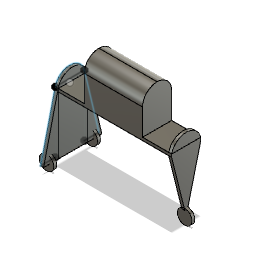
test_3 v2 (Autodesk Fusion 360 design; units mm, degrees)
part number: Configuration 1
Autodesk Fusion 360 part; units mm, degrees
sketch "Sketch1" plane through (0, 0, 0) normal (0, 0, 1) x (1, 0, 0)
  line L0 (0, 0) -> (200, 0)
  line L1 (200, 0) -> (200, 100)
  line L2 (200, 100) -> (0, 100)
  line L3 (0, 100) -> (0, 0)
  dimension "d1" = 200
  dimension "d2" = 100
  constraint horizontal L0
  constraint vertical L1
  constraint horizontal L2
  constraint vertical L3
  constraint coincident L0.start L3.end
  measures "d1" distance of L0.start L0.end
  measures "d2" distance of L0.start L2.end
extrude "Extrude1" add sketch "Sketch1" along normal blind 100 makes body 1
move_body "Move1" bodies 1 to x (1, 0, 0) y (0, 1, 0) z (0, 0, 1) at (0, 200, 0)
sketch "Sketch2" plane through (200, 0, 0) normal (1, 0, 0) x (0, 0, -1)
  line L0 (0, 200) -> (0, 300)
  line L1 (0, 300) -> (-100, 300)
  line L2 (-100, 300) -> (-100, 200)
  line L3 (-100, 200) -> (0, 200)
  line L4 (-100, 300) -> (-120, 300)
  line L5 (-120, 300) -> (-120, 280)
  line L6 (-120, 280) -> (-100, 280)
  line L7 (-100, 280) -> (-100, 300)
  line L8 (0, 300) -> (20, 300)
  line L9 (20, 300) -> (20, 280)
  line L10 (20, 280) -> (0, 280)
  line L11 (0, 280) -> (0, 300)
  dimension "d5" = 20
  dimension "d6" = 20
  dimension "d7" = 20
  dimension "d8" = 20
  constraint horizontal L4
  constraint vertical L5
  constraint horizontal L6
  constraint vertical L7
  constraint coincident L1.end L2.start
  constraint horizontal L8
  constraint vertical L9
  constraint horizontal L10
  constraint vertical L11
  constraint coincident L0.end L1.start
  measures "d5" distance of L1.end L4.end
  measures "d6" distance of L1.end L6.end
  measures "d7" distance of L0.end L8.end
  measures "d8" distance of L0.end L10.end
sketch "Sketch3" plane through (200, 0, 0) normal (1, 0, 0) x (0, 0, -1)
  line L0 (0, 200) -> (0, 300)
  line L1 (0, 300) -> (-100, 300)
  line L2 (-100, 300) -> (-100, 200)
  line L3 (-100, 200) -> (0, 200)
  line L4 (-100, 200) -> (0, 200)
  line L5 (0, 200) -> (0, 210)
  line L6 (0, 210) -> (-100, 210)
  line L7 (-100, 210) -> (-100, 200)
  dimension "d11" = 100
  dimension "d12" = 10
  constraint horizontal L4
  constraint vertical L5
  constraint horizontal L6
  constraint vertical L7
  constraint coincident L2.end L3.start
  measures "d11" distance of L2.end L0.start
  measures "d12" distance of L2.end L6.end
extrude "Extrude3" add sketch "Sketch3" along normal blind 100 separate body contours L0 L2 L3 L4 L5 L6 L7 makes body 2
copy_body "CopyPasteBodies1" bodies 2 makes body 3
move_body "Move2" bodies 3 to x (1, 0, 0) y (0, 1, 0) z (0, 0, 1) at (-300, 0, 0)
sketch "Sketch4" plane through (0, 200, 0) normal (0, -1, 0) x (1, 0, 0)
  line L0 (0, 0) -> (200, 0)
  line L1 (200, 0) -> (200, 100)
  line L2 (200, 100) -> (0, 100)
  line L3 (0, 100) -> (0, 0)
  line L4 (-100, 100) -> (-90, 100)
  line L5 (-90, 100) -> (-90, 0)
  line L6 (-90, 0) -> (-100, 0)
  line L7 (-100, 0) -> (-100, 100)
  constraint horizontal L4
  constraint vertical L5
  constraint horizontal L6
  constraint vertical L7
extrude "Extrude4" add sketch "Sketch4" along normal blind 200 contours L4 L5 L6 L7 bodies 3
sketch "Sketch5" plane through (-100, 0, 0) normal (-1, 0, 0) x (0, 0, 1)
  line L0 (100, 0) -> (100, 210)
  line L1 (100, 210) -> (0, 210)
  line L2 (0, 210) -> (0, 0)
  line L3 (0, 0) -> (100, 0)
  line L4 (100, 210) -> (150, 0)
  line L5 (150, 0) -> (100, 0)
  line L6 (100, 210) -> (0, 210)
  line L7 (0, 0) -> (-50, 0)
  line L8 (-50, 0) -> (0, 210)
  arc A0 (100, 210) -> (0, 210) centre (50, 198.0952) ccw
  constraint coincident L0.end L1.start
  constraint coincident L0.start L3.end
  constraint perpendicular L0 L5
  constraint coincident L1.end L2.start
  constraint coincident L2.end L3.start
  constraint perpendicular L2 L7
  constraint tangent L4 A0
extrude "Extrude5" add sketch "Sketch5" against normal blind 10 separate body contours L1 L6 A0 makes body 4
extrude "Extrude6" add sketch "Sketch5" against normal blind 10 separate body contours L0 L4 L5 | L2 L7 L8 makes body 5 at (-100, 70, 116.6667) makes body 6 at (-100, 70, -16.6667)
copy_body "CopyPasteBodies2" bodies 4 makes body 7
move_body "Move3" bodies 7 to x (1, 0, 0) y (0, 1, 0) z (0, 0, 1) at (390, 0, 0)
sketch "Sketch6" plane through (300, 0, 0) normal (1, 0, 0) x (0, 0, -1)
  arc A0 (0, 210) -> (-100, 210) centre (-50, 198.0952) ccw
  line L0 (-100, 210) -> (0, 210)
  line L1 (0, 200) -> (-100, 200)
  line L2 (-100, 200) -> (-50, 0)
  line L3 (-50, 0) -> (0, 200)
  constraint parallel L0 L1
extrude "Extrude7" add sketch "Sketch6" against normal blind 10 contours L1 L2 L3 bodies 2
sketch "Sketch7" plane through (300, 0, 0) normal (1, 0, 0) x (0, 0, -1)
  line L0 (-100, 210) -> (-100, 200)
  line L1 (-100, 200) -> (-50, 0)
  line L2 (-50, 0) -> (0, 200)
  line L3 (0, 200) -> (0, 210)
  line L4 (0, 210) -> (-100, 210)
  line L5 (-25, 0) -> (-75, 0)
  line L6 (-75, 0) -> (-75, 20)
  line L7 (-75, 20) -> (-25, 20)
  line L8 (-25, 20) -> (-25, 0)
  constraint horizontal L5
  constraint vertical L6
  constraint horizontal L7
  constraint vertical L8
extrude "Extrude8" cut sketch "Sketch7" against normal blind 20 contours L1 L2 L7 | L1 L5 L6 L7 | L2 L5 L7 L8 bodies 2
sketch "Sketch8" plane through (0, 0, 0) normal (0, 0, -1) x (-1, 0, 0)
  line L0 (0, 200) -> (0, 300)
  line L1 (0, 300) -> (-200, 300)
  line L2 (-200, 300) -> (-200, 200)
  line L3 (-200, 200) -> (0, 200)
  circle A0 centre (100, 0) radius 25
  point P0 (100, 0)
  dimension "d25" = 50
  measures "d25" diameter of A0
extrude "Extrude9" add sketch "Sketch8" along normal blind 10 separate body contours A0 makes body 8
move_body "Move4" bodies 8 to x (1, 0, 0) y (0, 1, 0) z (0, 0, 1) at (0, 0, -20)
copy_body "CopyPasteBodies3" bodies 8 makes body 9
move_body "Move5" bodies 9 to x (1, 0, 0) y (0, 1, 0) z (0, 0, 1) at (0, 0, 150)
copy_body "CopyPasteBodies4" bodies 8 makes body 10
move_body "Move6" bodies 10 to x (1, 0, 0) y (0, 1, 0) z (0, 0, 1) at (400, 0, 0)
move_body "Move7" bodies 10 to x (1, 0, 0) y (0, 1, 0) z (0, 0, 1) at (0, 0.9786, 75.2394)
fillet "Fillet1" radius 50 tangency weight 0.98939 2 edges at (100, 300, 0) (100, 300, 100) on bodies 1
move_body "Move8" bodies 1 to x (1, 0, 0) y (0, 1, 0) z (0, 0, 1) at (0, 50, 0)
extrude "Extrude10" add 1 faces at (66.6667, 250, 33.3333) along direction (0, -1, 0) blind 50 on bodies 1 bodies 1 4 5 6 7 8 9 10 2 3
